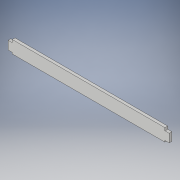
# Autodesk Inventor part: BB Gun Support
Saved by Autodesk Inventor 2018 (Build 220112000, 112)
## iProperties
Created: 2019-05-24
Part Number: BB Gun Support
Material: Generic
Document SubType Name: Modeling
Designer: 871357
Density: 1 g/cm^3
Appearance: Default
Author: 871357
Autodesk Inventor part; units mm, degrees
ref_plane "YZ Plane" through (0, 0, 0) normal (1, 0, 0) x (0, 1, 0)
ref_plane "XZ Plane" through (0, 0, 0) normal (0, 1, 0) x (-1, 0, 0)
ref_plane "XY Plane" through (0, 0, 0) normal (0, 0, 1) x (1, 0, 0)
sketch "Sketch1" plane through (0, 0, 0) normal (0, 0, 1) x (1, 0, 0)
  line L0 (0, 0) -> (139.7, 0)
  line L1 (139.7, 0) -> (139.7, 11.43)
  line L2 (139.7, 11.43) -> (0, 11.43)
  line L3 (0, 11.43) -> (0, 0)
  line L4 (0, 1.27) -> (-3.81, 1.27)
  line L5 (-3.81, 1.27) -> (-3.81, 8.89)
  line L6 (-3.81, 8.89) -> (0, 8.89)
  line L7 (0, 8.89) -> (0, 1.27)
  line L8 (139.7, 1.27) -> (143.51, 1.27)
  line L9 (143.51, 1.27) -> (143.51, 8.89)
  line L10 (143.51, 8.89) -> (139.7, 8.89)
  line L11 (139.7, 8.89) -> (139.7, 1.27)
  dimension "d0" = 139.7
  dimension "d1" = 11.43
  dimension "d2" = 3.81
  dimension "d3" = 7.62
  dimension "d4" = 1.27
  dimension "d5" = 3.81
  dimension "d6" = 7.62
  dimension "d7" = 1.27
  constraints: 24 end point, 6 parallel, 3 horizontal, 3 perpendicular, 2 point on line
  measures "d0" distance of L2.end L1.end
  measures "d1" distance of L2.end L0.start
  measures "d2" distance of L5.end L6.end
  measures "d3" distance of L4.end L5.end
  measures "d4" distance between parallel lines of L0 L4
  measures "d5" distance of L10.end L9.end
  measures "d6" distance of L9.end L8.end
  measures "d7" distance between parallel lines of L0 L8
extrude "Extrusion1" add sketch "Sketch1" along normal blind 2.54
body "Solid1"
